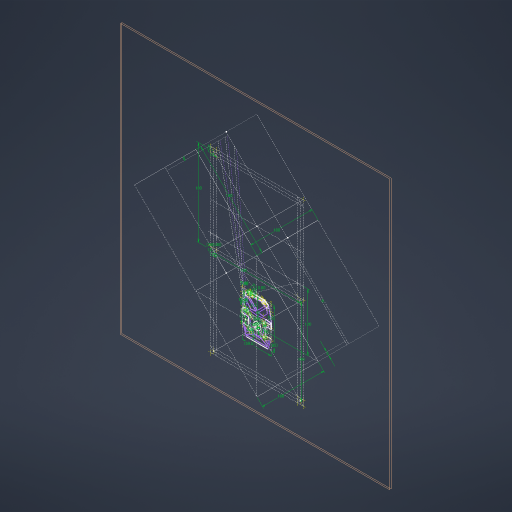
# Autodesk Inventor part: chassis
Saved by Autodesk Inventor 2023.5 (Build 275446000, 446)
## iProperties
Created: 2024-12-08
Part Number: chassis
Material: 一般
Document SubType Name: Modeling
Designer: IshiiLabHonda
Density: 1 g/cm^3
Appearance: 既定
Author: IshiiLabHonda
Autodesk Inventor part; units mm, degrees
(part 1 of 2)
ref_plane "YZ Plane" through (0, 0, 0) normal (1, 0, 0) x (0, 1, 0)
ref_plane "XZ Plane" through (0, 0, 0) normal (0, 1, 0) x (-1, 0, 0)
sketch "スケッチ1" plane through (0, 0, 0) normal (0, 0, 1) x (1, 0, 0)
  line L0 (0, 0) -> (0, 1) construction
  line L1 (0, 0) -> (1, 0) construction
  line L2 (-90, 90) -> (90, 90) construction
  line L3 (90, 90) -> (90, -90) construction
  line L4 (90, -90) -> (-90, -90) construction
  line L5 (-90, -90) -> (-90, 90) construction
  line L6 (-90, -90) -> (90, 90) construction
  line L7 (-90, 90) -> (90, -90) construction
  line L8 (-84, 96) -> (-84, 84) construction
  line L9 (-84, 84) -> (-96, 84) construction
  line L10 (-96, 84) -> (-96, 96) construction
  line L11 (-96, 96) -> (-84, 84) construction
  line L12 (-84, 96) -> (-96, 84) construction
  line L13 (-96, 96) -> (-84, 96) construction
  line L14 (-96, -96) -> (-96, -84) construction
  line L15 (-84, -96) -> (-96, -96) construction
  line L16 (-96, -96) -> (-84, -84) construction
  line L17 (-96, -84) -> (-84, -96) construction
  line L18 (-84, -84) -> (-84, -96) construction
  line L19 (-96, -84) -> (-84, -84) construction
  line L20 (96, -96) -> (84, -96) construction
  line L21 (96, -84) -> (96, -96) construction
  line L22 (96, -96) -> (84, -84) construction
  line L23 (84, -96) -> (96, -84) construction
  line L24 (84, -84) -> (96, -84) construction
  line L25 (84, -96) -> (84, -84) construction
  line L26 (96, 96) -> (96, 84) construction
  line L27 (84, 96) -> (96, 96) construction
  line L28 (96, 96) -> (84, 84) construction
  line L29 (96, 84) -> (84, 96) construction
  line L30 (84, 84) -> (84, 96) construction
  line L31 (96, 84) -> (84, 84) construction
  line L32 (-84, 84) -> (-84, -84) construction
  line L33 (-96, 84) -> (-96, -84) construction
  line L34 (-84, -84) -> (84, -84) construction
  line L35 (-84, -96) -> (84, -96) construction
  line L36 (96, 84) -> (96, -84) construction
  line L37 (84, 84) -> (84, -84) construction
  line L38 (-84, 96) -> (84, 96) construction
  line L39 (-84, 84) -> (84, 84) construction
  line L40 (-18, 15) -> (18, 15) construction
  line L41 (18, 15) -> (18, -15) construction
  line L42 (18, -15) -> (-18, -15) construction
  line L43 (-18, -15) -> (-18, 15) construction
  line L44 (-18, 15) -> (18, -15) construction
  line L45 (18, 15) -> (-18, -15) construction
  line L46 (-29.25, 11.5) -> (-18, 11.5) construction
  line L47 (-18, -11.5) -> (-29.25, -11.5) construction
  line L48 (-29.25, -11.5) -> (-29.25, 11.5) construction
  line L49 (-29.25, 11.5) -> (-18, -11.5) construction
  line L50 (-18, 11.5) -> (-29.25, -11.5) construction
  line L51 (29.25, 11.5) -> (18, 11.5) construction
  line L52 (18, -11.5) -> (29.25, -11.5) construction
  line L53 (29.25, -11.5) -> (29.25, 11.5) construction
  line L54 (29.25, 11.5) -> (18, -11.5) construction
  line L55 (18, 11.5) -> (29.25, -11.5) construction
  line L56 (-18, -10) -> (18, -10) construction
  line L57 (-18, -12.5) -> (18, -12.5) construction
  line L58 (-18, 10) -> (18, 10) construction
  line L59 (-18, 12.5) -> (18, 12.5) construction
  line L60 (-16, -15) -> (-16, 15) construction
  line L61 (16, -15) -> (16, 15) construction
  line L62 (-12, -10) -> (-12, -15) construction
  line L63 (-16, -10) -> (-12, -15) construction
  line L64 (-16, -15) -> (-12, -10) construction
  circle A0 centre (-14, -12.5) radius 0.8 construction
  line L65 (12, -10) -> (12, -15) construction
  line L66 (16, -10) -> (12, -15) construction
  line L67 (16, -15) -> (12, -10) construction
  circle A1 centre (14, -12.5) radius 0.8 construction
  line L68 (-12, 10) -> (-12, 15) construction
  line L69 (-16, 10) -> (-12, 15) construction
  line L70 (-16, 15) -> (-12, 10) construction
  circle A2 centre (-14, 12.5) radius 0.8 construction
  line L71 (12, 10) -> (12, 15) construction
  line L72 (16, 10) -> (12, 15) construction
  circle A3 centre (14, 12.5) radius 0.8 construction
  line L73 (16, 15) -> (12, 10) construction
  line L74 (-96, 276) -> (-84, 276) construction
  line L75 (-84, 276) -> (-84, 264) construction
  line L76 (-84, 264) -> (-96, 264) construction
  line L77 (-96, 264) -> (-96, 276) construction
  line L78 (-96, 276) -> (-84, 264) construction
  line L79 (-84, 276) -> (-96, 264) construction
  line L80 (-90, 90) -> (-90, 270) construction
  line L81 (-96, 264) -> (-96, 96) construction
  line L82 (-84, 264) -> (-84, 96) construction
  line L83 (96, 276) -> (84, 276) construction
  line L84 (84, 276) -> (84, 264) construction
  line L85 (84, 264) -> (96, 264) construction
  line L86 (96, 264) -> (96, 276) construction
  line L87 (96, 276) -> (84, 264) construction
  line L88 (84, 276) -> (96, 264) construction
  line L89 (90, 90) -> (90, 270) construction
  line L90 (96, 264) -> (96, 96) construction
  line L91 (84, 264) -> (84, 96) construction
  line L92 (-84, 276) -> (84, 276) construction
  line L93 (-84, 264) -> (84, 264) construction
  line L94 (-90, 270) -> (90, 270) construction
  line L95 (-90, 270) -> (90, 90) construction
  line L96 (-90, 90) -> (90, 270) construction
  circle A4 centre (0, 0) radius 15 construction
  line L97 (-96, 120) -> (96, 120) construction
  line L98 (0, 127.2792) -> (0, -127.2792) construction
  line L99 (-127.2792, 0) -> (127.2792, 0) construction
  line L100 (127.2792, 0) -> (0, -127.2792) construction
  line L101 (0, -127.2792) -> (-127.2792, 0) construction
  line L102 (-127.2792, 0) -> (0, 127.2792) construction
  line L103 (0, 127.2792) -> (127.2792, 0) construction
  line L104 (127.2792, 254.5584) -> (254.5584, 127.2792) construction
  line L105 (254.5584, 127.2792) -> (127.2792, 0) construction
  line L106 (127.2792, 0) -> (0, 127.2792) construction
  line L107 (0, 127.2792) -> (127.2792, 254.5584) construction
  line L108 (-127.2792, 254.5584) -> (0, 127.2792) construction
  line L109 (0, 127.2792) -> (-127.2792, 0) construction
  line L110 (-127.2792, 0) -> (-254.5584, 127.2792) construction
  line L111 (-254.5584, 127.2792) -> (-127.2792, 254.5584) construction
  line L112 (0, 381.8377) -> (127.2792, 254.5584) construction
  line L113 (127.2792, 254.5584) -> (0, 127.2792) construction
  line L114 (0, 127.2792) -> (-127.2792, 254.5584) construction
  line L115 (-127.2792, 254.5584) -> (0, 381.8377) construction
  line L116 (190.9188, 63.6396) -> (63.6396, 190.9188) construction
  line L117 (-190.9188, 190.9188) -> (-63.6396, 63.6396) construction
  line L118 (59.397, -59.397) -> (186.6762, 67.8823) construction
  line L119 (59.397, 186.6762) -> (186.6762, 59.397) construction
  line L120 (63.6396, 190.9188) -> (-63.6396, 318.1981) construction
  line L121 (-186.6762, 186.6762) -> (-59.397, 313.9554) construction
  point P0 (-90, -90)
  point P1 (90, -90)
  point P2 (-23.625, 0)
  point P3 (-84, 120)
  point P4 (84, 120)
  point P5 (0, 0)
  dimension "d0" = 1
  dimension "d1" = 1
  dimension "d2" = 180
  dimension "d3" = 180
  dimension "d4" = 12
  dimension "d5" = 12
  dimension "d8" = 360
  dimension "d10" = 36
  dimension "d12" = 11.25
  dimension "d13" = 23
  dimension "d14" = 5
  dimension "d15" = 2
  dimension "d16" = 4
  dimension "d17" = 1.6
  dimension "d22" = 12
  dimension "d23" = 12
  dimension "d24" = 180
  dimension "d25" = 25
  dimension "d26" = 30
  dimension "d27" = 30
  dimension "d29" = 120
  dimension "d331" = 180
  dimension "d334" = 180
  dimension "d337" = 180
  dimension "d340" = 6
  dimension "d341" = 6
  dimension "d342" = 6
  constraints: 244 end point, 29 point on line, 27 symmetric about line, 19 midpoint, 18 parallel, 10 perpendicular, 5 centre point, 4 coincident, 2 collinear, 1 horizontal, 1 vertical, 91 other
  measures "d0" distance of L0.start L0.end
  measures "d1" distance of L0.start L1.end
  measures "d2" distance of L2.start L2.end
  measures "d3" distance of L2.end L3.end
  measures "d4" distance of L9.end L10.end
  measures "d5" distance of L8.end L9.end
  measures "d10" distance of L40.start L40.end
  measures "d12" distance of L46.start L46.end
  measures "d13" distance of L47.end L46.start
  measures "d14" distance between parallel lines of L56 L42
  measures "d15" distance between parallel lines of L43 L60
  measures "d16" distance between parallel lines of L60 L62
  measures "d17" diameter of A0
  measures "d22" distance of L75.end L76.end
  measures "d23" distance of L76.end L74.start
  measures "d24" distance of L2.start L80.end
  measures "d25" distance between parallel lines of L57 L59
  measures "d26" distance between parallel lines of L42 L40
  measures "d27" diameter of A4
  measures "d29" distance between parallel lines of L1 L97
  measures "d331" distance of L100.start L100.end
  measures "d334" distance of L102.end L104.start
  measures "d337" distance of L102.end L108.start
  measures "d340" distance between parallel lines of L118 L105
  measures "d341" distance between parallel lines of L116 L119
  measures "d342" distance between parallel lines of L111 L121
sketch "スケッチ4" plane through (0, 0, 0) normal (0, 0, 1) x (1, 0, 0)
  line L0 (-84, 264) -> (-96, 264) construction
  line L1 (-90, 90) -> (-90, 270) construction
  line L2 (-96, 264) -> (-96, 96) construction
  line L3 (-96, 96) -> (-84, 96) construction
  line L4 (-84, 96) -> (-84, 84) construction
  line L5 (-84, 96) -> (-96, 84) construction
  line L6 (-96, 96) -> (-84, 84) construction
  line L7 (-84, 264) -> (-84, 96) construction
  line L8 (-84, 84) -> (-96, 84) construction
  line L9 (84, -84) -> (96, -84) construction
  line L10 (84, -96) -> (96, -84) construction
  line L11 (96, -96) -> (84, -84) construction
  line L12 (96, -84) -> (96, -96) construction
  line L13 (96, -96) -> (84, -96) construction
  line L14 (0, 0) -> (0, 1) construction
  line L15 (0, 0) -> (1, 0) construction
  line L16 (16, 15) -> (12, 10) construction
  line L17 (-96, 84) -> (-96, -84) construction
  line L18 (-84, 84) -> (-84, -84) construction
  line L19 (-90, -90) -> (-90, 90) construction
  line L20 (-90, 90) -> (90, 90) construction
  line L21 (-84, -84) -> (84, -84) construction
  line L22 (-84, -96) -> (84, -96) construction
  line L23 (-90, -90) -> (90, 90) construction
  line L24 (90, -90) -> (-90, -90) construction
  line L25 (-90, 90) -> (90, -90) construction
  line L26 (84, 84) -> (84, -84) construction
  line L27 (90, 90) -> (90, -90) construction
  line L28 (96, 84) -> (96, -84) construction
  line L29 (-96, 84) -> (-96, 96) construction
  line L30 (-84, -84) -> (-84, -96) construction
  line L31 (-96, -84) -> (-84, -84) construction
  line L32 (-84, -96) -> (-96, -96) construction
  line L33 (-96, -96) -> (-84, -84) construction
  line L34 (-96, -84) -> (-84, -96) construction
  line L35 (-96, -96) -> (-96, -84) construction
  line L36 (84, -96) -> (84, -84) construction
  line L37 (-18, -15) -> (-18, 15) construction
  line L38 (-29.25, 11.5) -> (-18, 11.5) construction
  line L39 (-18, -11.5) -> (-29.25, -11.5) construction
  line L40 (-18, 11.5) -> (-29.25, -11.5) construction
  line L41 (-29.25, 11.5) -> (-18, -11.5) construction
  line L42 (-29.25, -11.5) -> (-29.25, 11.5) construction
  line L43 (12, 10) -> (12, 15) construction
  circle A0 centre (14, 12.5) radius 0.8 construction
  line L44 (29.25, 11.5) -> (18, 11.5) construction
  line L45 (16, 10) -> (12, 15) construction
  circle A1 centre (14, -12.5) radius 0.8 construction
  line L46 (16, -15) -> (12, -10) construction
  line L47 (16, -10) -> (12, -15) construction
  line L48 (12, -10) -> (12, -15) construction
  circle A2 centre (-14, -12.5) radius 0.8 construction
  line L49 (-12, -10) -> (-12, -15) construction
  line L50 (-16, -15) -> (-12, -10) construction
  line L51 (-16, -10) -> (-12, -15) construction
  line L52 (96, 84) -> (84, 84) construction
  line L53 (96, 96) -> (96, 84) construction
  line L54 (84, 96) -> (96, 96) construction
  line L55 (96, 96) -> (84, 84) construction
  line L56 (84, 84) -> (84, 96) construction
  line L57 (96, 84) -> (84, 96) construction
  line L58 (-96, 264) -> (-96, 276) construction
  line L59 (-84, 276) -> (-84, 264) construction
  line L60 (-96, 276) -> (-84, 276) construction
  line L61 (-96, 276) -> (-84, 264) construction
  line L62 (-84, 276) -> (-96, 264) construction
  line L63 (-84, 84) -> (84, 84) construction
  line L64 (-84, 96) -> (84, 96) construction
  line L65 (84, 264) -> (84, 96) construction
  line L66 (90, 90) -> (90, 270) construction
  line L67 (-90, 90) -> (90, 270) construction
  line L68 (-90, 270) -> (90, 90) construction
  line L69 (96, 264) -> (96, 96) construction
  line L70 (-96, 120) -> (96, 120) construction
  line L71 (-84, 264) -> (84, 264) construction
  line L72 (-84, 276) -> (84, 276) construction
  line L73 (-90, 270) -> (90, 270) construction
  line L74 (84, 276) -> (84, 264) construction
  line L75 (84, 264) -> (96, 264) construction
  line L76 (96, 264) -> (96, 276) construction
  line L77 (96, 276) -> (84, 264) construction
  line L78 (96, 276) -> (84, 276) construction
  line L79 (84, 276) -> (96, 264) construction
  line L80 (-18, 15) -> (18, 15) construction
  line L81 (18, 15) -> (18, -15) construction
  line L82 (18, -15) -> (-18, -15) construction
  circle A3 centre (-14, 12.5) radius 0.8 construction
  line L83 (-16, 10) -> (-12, 15) construction
  line L84 (-12, 10) -> (-12, 15) construction
  line L85 (-16, 15) -> (-12, 10) construction
  circle A4 centre (0, 0) radius 15 construction
  line L86 (-18, 10) -> (18, 10) construction
  line L87 (-18, 12.5) -> (18, 12.5) construction
  line L88 (-18, 15) -> (18, -15) construction
  line L89 (18, 15) -> (-18, -15) construction
  line L90 (-18, -10) -> (18, -10) construction
  line L91 (-18, -12.5) -> (18, -12.5) construction
  line L92 (16, -15) -> (16, 15) construction
  line L93 (18, 11.5) -> (29.25, -11.5) construction
  line L94 (18, -11.5) -> (29.25, -11.5) construction
  line L95 (29.25, -11.5) -> (29.25, 11.5) construction
  line L96 (29.25, 11.5) -> (18, -11.5) construction
  line L97 (-16, -15) -> (-16, 15) construction
  line L98 (-84, 120) -> (29.25, 40.7015) construction
  line L99 (84, 120) -> (-29.25, 40.7015) construction
  line L100 (-29.25, 55) -> (29.25, 55) construction
  line L101 (-1.8558, 55) -> (-29.25, 35.8184) construction
  line L102 (1.8558, 55) -> (29.25, 35.8184) construction
  line L103 (-15.8034, 55) -> (-29.25, 45.5846) construction
  line L104 (-13.0898, 56.2897) -> (-9.0748, 50.5556) construction
  line L105 (-9.0748, 50.5556) -> (-14.3993, 46.8274) construction
  line L106 (-14.3993, 46.8274) -> (-18.4143, 52.5615) construction
  line L107 (-18.4143, 52.5615) -> (-13.0898, 56.2897) construction
  line L108 (-13.0898, 56.2897) -> (-14.3993, 46.8274) construction
  line L109 (-9.0748, 50.5556) -> (-18.4143, 52.5615) construction
  line L110 (-12.5162, 55.4705) -> (-17.8407, 51.7423) construction
  line L111 (-9.6483, 51.3748) -> (-14.9728, 47.6465) construction
  line L112 (-13.7445, 51.5585) -> (-13.0892, 52.0174) construction
  line L113 (-13.7445, 51.5585) -> (-13.2857, 50.9032) construction
  line L114 (-13.3762, 53.6476) -> (-11.6554, 51.1902) construction
  line L115 (-11.6554, 51.1902) -> (-14.1129, 49.4694) construction
  line L116 (-14.1129, 49.4694) -> (-15.8336, 51.9269) construction
  line L117 (-15.8336, 51.9269) -> (-13.3762, 53.6476) construction
  line L118 (-13.3762, 53.6476) -> (-14.1129, 49.4694) construction
  line L119 (-11.6554, 51.1902) -> (-15.8336, 51.9269) construction
  circle A5 centre (-13.7445, 51.5585) radius 0.8 construction
  line L120 (-29.25, 11.5) -> (-29.25, 55) construction
  line L121 (29.25, 11.5) -> (29.25, 55) construction
  line L122 (-8.9966, 50) -> (8.9966, 50) construction
  line L123 (-29.75, 55) -> (-29.75, -30) construction
  line L124 (29.75, 55) -> (29.75, -30) construction
  line L125 (-29.25, 55) -> (-29.75, 55) construction
  line L126 (29.25, 55) -> (29.75, 55) construction
  line L127 (-29.75, 8.5) -> (29.75, 8.5) construction
  line L128 (-29.75, -8.5) -> (29.75, -8.5) construction
  circle A6 centre (0, 0) radius 7.5 construction
  line L129 (-29.75, -30) -> (29.75, -30) construction
  line L130 (-29.25, 45.5846) -> (-29.75, 45.2345) construction
  line L131 (-29.25, 35.8184) -> (-29.75, 35.4683) construction
  line L132 (-25.25, 18.5) -> (-25.3613, 19.2922) construction
  line L133 (-25.25, 18.5) -> (-24.4578, 18.6113) construction
  line L134 (-28.0736, 20.6277) -> (-23.1223, 21.3236) construction
  line L135 (-23.1223, 21.3236) -> (-22.4264, 16.3723) construction
  line L136 (-22.4264, 16.3723) -> (-27.3777, 15.6764) construction
  line L137 (-27.3777, 15.6764) -> (-28.0736, 20.6277) construction
  line L138 (-28.0736, 20.6277) -> (-22.4264, 16.3723) construction
  line L139 (-23.1223, 21.3236) -> (-27.3777, 15.6764) construction
  circle A7 centre (-25.25, 18.5) radius 0.8 construction
  line L140 (-25.25, 55) -> (-25.25, -30) construction
  line L141 (-96, 180) -> (96, 180) construction
  line L142 (-25.3613, 19.2922) -> (-65.8646, 307.4878) construction
  line L143 (-186.6762, 186.6762) -> (-59.397, 313.9554) construction
  line L144 (59.397, 186.6762) -> (186.6762, 59.397) construction
  line L145 (-25.25, 18.5) -> (-80.9717, 292.3807) construction
  line L146 (-25.25, 18.5) -> (-47.5722, 302.1307) construction
  line L147 (63.6396, 190.9188) -> (-63.6396, 318.1981) construction
  line L148 (13.0898, 56.2897) -> (9.0748, 50.5556) construction
  line L149 (9.0748, 50.5556) -> (14.3993, 46.8274) construction
  line L150 (14.3993, 46.8274) -> (18.4143, 52.5615) construction
  line L151 (18.4143, 52.5615) -> (13.0898, 56.2897) construction
  line L152 (13.0898, 56.2897) -> (14.3993, 46.8274) construction
  line L153 (9.0748, 50.5556) -> (18.4143, 52.5615) construction
  line L154 (12.5162, 55.4705) -> (17.8407, 51.7423) construction
  line L155 (9.6483, 51.3748) -> (14.9728, 47.6465) construction
  line L156 (13.7445, 51.5585) -> (13.0892, 52.0174) construction
  line L157 (13.7445, 51.5585) -> (13.2857, 50.9032) construction
  line L158 (13.3762, 53.6476) -> (11.6554, 51.1902) construction
  line L159 (11.6554, 51.1902) -> (14.1129, 49.4694) construction
  line L160 (14.1129, 49.4694) -> (15.8336, 51.9269) construction
  line L161 (15.8336, 51.9269) -> (13.3762, 53.6476) construction
  line L162 (13.3762, 53.6476) -> (14.1129, 49.4694) construction
  line L163 (11.6554, 51.1902) -> (15.8336, 51.9269) construction
  circle A8 centre (13.7445, 51.5585) radius 0.8 construction
  line L164 (-23.1223, 21.3236) -> (-18.1709, 22.0195) construction
  line L165 (-18.1709, 22.0195) -> (-17.4751, 17.0681) construction
  line L166 (-17.4751, 17.0681) -> (-22.4264, 16.3723) construction
  line L167 (-23.1223, 21.3236) -> (-28.0736, 20.6277) construction
  line L168 (-28.0736, 20.6277) -> (-27.3777, 15.6764) construction
  line L169 (-27.3777, 15.6764) -> (-22.4264, 16.3723) construction
  line L170 (27.3777, 15.6764) -> (28.0736, 20.6277) construction
  line L171 (23.1223, 21.3236) -> (18.1709, 22.0195) construction
  line L172 (18.1709, 22.0195) -> (17.4751, 17.0681) construction
  line L173 (17.4751, 17.0681) -> (22.4264, 16.3723) construction
  line L174 (23.1223, 21.3236) -> (28.0736, 20.6277) construction
  line L175 (28.0736, 20.6277) -> (27.3777, 15.6764) construction
  line L176 (27.3777, 15.6764) -> (22.4264, 16.3723) construction
  line L177 (23.1223, 21.3236) -> (27.3777, 15.6764) construction
  line L178 (22.4264, 16.3723) -> (28.0736, 20.6277) construction
  line L179 (-20.2987, 19.1959) -> (-61.4376, 311.9148) construction
  line L180 (-20.2987, 19.1959) -> (-76.7397, 296.6126) construction
  line L181 (-20.2987, 19.1959) -> (-42.1385, 296.6969) construction
  line L182 (-23.1223, 21.3236) -> (-17.4751, 17.0681) construction
  line L183 (-22.4264, 16.3723) -> (-18.1709, 22.0195) construction
  point P0 (90, -90)
  point P1 (-90, -90)
  point P2 (-23.625, 0)
  point P3 (0, 61.1826)
  point P4 (-8.8296, 55)
  point P5 (-11.0823, 53.4227)
  point P6 (0, 180)
  point P7 (11.0823, 53.4227)
  dimension "d264" = 110
  dimension "d275" = 7
  dimension "d276" = 6.5
  dimension "d277" = 5
  dimension "d278" = 3
  dimension "d279" = 3
  dimension "d280" = 1.6
  dimension "d281" = 8
  dimension "d284" = 5
  dimension "d288" = 17
  dimension "d289" = 15
  dimension "d290" = 0.5
  dimension "d291" = 0.5
  dimension "d292" = 85
  dimension "d296" = 5
  dimension "d297" = 5
  dimension "d298" = 1.6
  dimension "d299" = 8
  dimension "d345" = 7
  dimension "d346" = 7
  dimension "d356" = 15
  dimension "d367" = 4
  dimension "d369" = 40
  dimension "d370" = 6
  dimension "d371" = 59.5
  dimension "d382" = 5
  dimension "d385" = 7
  constraints: 166 end point, 38 point on line, 25 symmetric about line, 18 parallel, 13 midpoint, 13 perpendicular, 6 point on circle, 5 collinear, 4 centre point, 4 coincident, 2 equal length, 8 other
  measures "d264" angle of L99 L98
  measures "d275" distance of L104.start L104.end
  measures "d276" distance of L106.end L104.start
  measures "d277" distance between parallel lines of L110 L111
  measures "d278" distance of L115.end L116.end
  measures "d279" distance of L114.end L115.end
  measures "d280" diameter of A5
  measures "d281" distance between parallel lines of L101 L103
  measures "d284" distance between parallel lines of L100 L122
  measures "d288" distance between parallel lines of L128 L127
  measures "d289" diameter of A6
  measures "d290" distance between parallel lines of L123 L120
  measures "d291" distance between parallel lines of L121 L124
  measures "d292" distance between parallel lines of L129 L100
  measures "d296" distance of L135.end L136.end
  measures "d297" distance of L134.end L135.end
  measures "d298" diameter of A7
  measures "d299" angle of L140 L132
  measures "d345" angle of L145 L146
  measures "d346" distance from line of L38 L132.start
  measures "d356" distance between parallel lines of L129 L82
  measures "d367" distance between parallel lines of L120 L140
  measures "d369" distance between parallel lines of L80 L100
  measures "d370" distance of L112.start point (-8.83, 55)
  measures "d371" distance of L123.end L124.end
  measures "d382" distance of L134.end L164.end
  measures "d385" angle of L180 L181
sketch "スケッチ5" plane through (0, 0, 0) normal (0, 0, 1) x (1, 0, 0)
  line L0 (0, 0) -> (0, 1) construction
  line L1 (29.25, 11.5) -> (18, 11.5) construction
  line L2 (18, 11.5) -> (29.25, -11.5) construction
  line L3 (29.25, 11.5) -> (18, -11.5) construction
  line L4 (29.25, -11.5) -> (29.25, 11.5) construction
  line L5 (18, -11.5) -> (29.25, -11.5) construction
  line L6 (-90, 90) -> (90, 90) construction
  line L7 (-90, -90) -> (90, 90) construction
  line L8 (-90, 90) -> (90, -90) construction
  line L9 (-84, 84) -> (-84, -84) construction
  line L10 (-96, 84) -> (-96, -84) construction
  line L11 (-90, -90) -> (-90, 90) construction
  line L12 (-84, 84) -> (-96, 84) construction
  line L13 (-96, 84) -> (-96, 96) construction
  line L14 (84, 84) -> (84, -84) construction
  line L15 (90, 90) -> (90, -90) construction
  line L16 (96, 84) -> (84, 84) construction
  line L17 (96, 84) -> (96, -84) construction
  line L18 (90, -90) -> (-90, -90) construction
  line L19 (-84, -84) -> (84, -84) construction
  line L20 (-84, -96) -> (84, -96) construction
  line L21 (-84, -84) -> (-84, -96) construction
  line L22 (-96, -96) -> (-96, -84) construction
  line L23 (-84, -96) -> (-96, -96) construction
  line L24 (-96, -96) -> (-84, -84) construction
  line L25 (-96, -84) -> (-84, -96) construction
  line L26 (-96, -84) -> (-84, -84) construction
  line L27 (0, 0) -> (1, 0) construction
  line L28 (-84, 264) -> (-96, 264) construction
  line L29 (-96, 276) -> (-84, 276) construction
  line L30 (-96, 264) -> (-96, 276) construction
  line L31 (-84, 276) -> (-96, 264) construction
  line L32 (-96, 276) -> (-84, 264) construction
  line L33 (-84, 276) -> (-84, 264) construction
  line L34 (84, -96) -> (84, -84) construction
  line L35 (96, -96) -> (84, -96) construction
  line L36 (96, -84) -> (96, -96) construction
  line L37 (96, -96) -> (84, -84) construction
  line L38 (84, -96) -> (96, -84) construction
  line L39 (84, -84) -> (96, -84) construction
  line L40 (-18, 15) -> (18, 15) construction
  line L41 (18, 15) -> (18, -15) construction
  line L42 (16, 15) -> (12, 10) construction
  line L43 (12, 10) -> (12, 15) construction
  line L44 (16, 10) -> (12, 15) construction
  line L45 (16, -15) -> (16, 15) construction
  line L46 (-18, 10) -> (18, 10) construction
  line L47 (-18, 12.5) -> (18, 12.5) construction
  circle A0 centre (0, 0) radius 15 construction
  line L48 (-18, -10) -> (18, -10) construction
  line L49 (-18, -12.5) -> (18, -12.5) construction
  line L50 (18, -15) -> (-18, -15) construction
  line L51 (-18, 15) -> (18, -15) construction
  line L52 (18, 15) -> (-18, -15) construction
  line L53 (-16, -15) -> (-16, 15) construction
  line L54 (-18, -15) -> (-18, 15) construction
  line L55 (-29.25, 11.5) -> (-18, 11.5) construction
  line L56 (-18, -11.5) -> (-29.25, -11.5) construction
  line L57 (-29.25, -11.5) -> (-29.25, 11.5) construction
  line L58 (-29.25, 11.5) -> (-18, -11.5) construction
  line L59 (-18, 11.5) -> (-29.25, -11.5) construction
  line L60 (-12, 10) -> (-12, 15) construction
  circle A1 centre (-14, 12.5) radius 0.8 construction
  line L61 (-16, 10) -> (-12, 15) construction
  line L62 (-16, 15) -> (-12, 10) construction
  circle A2 centre (14, 12.5) radius 0.8 construction
  line L63 (-84, 96) -> (-96, 84) construction
  line L64 (-96, 96) -> (-84, 96) construction
  line L65 (-84, 96) -> (-84, 84) construction
  line L66 (-96, 96) -> (-84, 84) construction
  line L67 (-96, 264) -> (-96, 96) construction
  line L68 (-84, 264) -> (-84, 96) construction
  line L69 (-84, 96) -> (84, 96) construction
  line L70 (-84, 84) -> (84, 84) construction
  line L71 (84, 84) -> (84, 96) construction
  line L72 (96, 96) -> (96, 84) construction
  line L73 (96, 96) -> (84, 84) construction
  line L74 (96, 84) -> (84, 96) construction
  line L75 (-96, 120) -> (96, 120) construction
  line L76 (84, 96) -> (96, 96) construction
  line L77 (-84, 264) -> (84, 264) construction
  line L78 (84, 264) -> (84, 96) construction
  line L79 (-84, 276) -> (84, 276) construction
  line L80 (96, 264) -> (96, 96) construction
  line L81 (-90, 270) -> (90, 270) construction
  line L82 (-90, 270) -> (90, 90) construction
  line L83 (-90, 90) -> (90, 270) construction
  line L84 (90, 90) -> (90, 270) construction
  line L85 (-90, 90) -> (-90, 270) construction
  line L86 (84, 264) -> (96, 264) construction
  line L87 (96, 276) -> (84, 276) construction
  line L88 (96, 276) -> (84, 264) construction
  line L89 (84, 276) -> (96, 264) construction
  line L90 (96, 264) -> (96, 276) construction
  line L91 (84, 276) -> (84, 264) construction
  circle A3 centre (-14, -12.5) radius 0.8 construction
  line L92 (-12, -10) -> (-12, -15) construction
  line L93 (-16, -15) -> (-12, -10) construction
  line L94 (12, -10) -> (12, -15) construction
  circle A4 centre (14, -12.5) radius 0.8 construction
  line L95 (16, -15) -> (12, -10) construction
  line L96 (16, -10) -> (12, -15) construction
  line L97 (-16, -10) -> (-12, -15) construction
  line L98 (-15.8336, 51.9269) -> (-13.3762, 53.6476) construction
  line L99 (-11.6554, 51.1902) -> (-15.8336, 51.9269) construction
  circle A5 centre (-13.7445, 51.5585) radius 0.8 construction
  line L100 (-11.6554, 51.1902) -> (-14.1129, 49.4694) construction
  line L101 (-13.3762, 53.6476) -> (-14.1129, 49.4694) construction
  line L102 (-14.1129, 49.4694) -> (-15.8336, 51.9269) construction
  line L103 (-29.25, 45.5846) -> (-29.75, 45.2345) construction
  line L104 (-15.8034, 55) -> (-29.25, 45.5846) construction
  line L105 (-29.25, 55) -> (-29.75, 55) construction
  line L106 (-13.3762, 53.6476) -> (-11.6554, 51.1902) construction
  line L107 (-29.25, 55) -> (29.25, 55) construction
  line L108 (-9.0748, 50.5556) -> (-14.3993, 46.8274) construction
  line L109 (-14.3993, 46.8274) -> (-18.4143, 52.5615) construction
  line L110 (-13.0898, 56.2897) -> (-9.0748, 50.5556) construction
  line L111 (-1.8558, 55) -> (-29.25, 35.8184) construction
  line L112 (1.8558, 55) -> (29.25, 35.8184) construction
  line L113 (-18, 15) -> (18, 15) construction
  line L114 (12, 10) -> (12, 15) construction
  line L115 (-18, 10) -> (18, 10) construction
  circle A6 centre (-14, 12.5) radius 0.8 construction
  line L116 (-12, 10) -> (-12, 15) construction
  line L117 (-16, 10) -> (-12, 15) construction
  line L118 (-16, 15) -> (-12, 10) construction
  line L119 (-18, 12.5) -> (18, 12.5) construction
  line L120 (29.25, 55) -> (29.75, 55) construction
  line L121 (29.25, 11.5) -> (29.25, 55) construction
  line L122 (-8.9966, 50) -> (8.9966, 50) construction
  line L123 (-29.25, 35.8184) -> (-29.75, 35.4683) construction
  line L124 (-29.25, 11.5) -> (-29.25, 55) construction
  line L125 (-9.6483, 51.3748) -> (-14.9728, 47.6465) construction
  line L126 (-13.7445, 51.5585) -> (-13.2857, 50.9032) construction
  line L127 (-13.7445, 51.5585) -> (-13.0892, 52.0174) construction
  line L128 (-9.0748, 50.5556) -> (-18.4143, 52.5615) construction
  line L129 (-12.5162, 55.4705) -> (-17.8407, 51.7423) construction
  line L130 (-18.4143, 52.5615) -> (-13.0898, 56.2897) construction
  line L131 (-13.0898, 56.2897) -> (-14.3993, 46.8274) construction
  line L132 (-29.25, 11.5) -> (-18, 11.5) construction
  line L133 (-29.25, 11.5) -> (-18, -11.5) construction
  line L134 (29.25, 11.5) -> (18, 11.5) construction
  line L135 (29.25, -11.5) -> (29.25, 11.5) construction
  line L136 (18, 11.5) -> (29.25, -11.5) construction
  line L137 (29.25, 11.5) -> (18, -11.5) construction
  line L138 (0, 0) -> (0, 1) construction
  line L139 (0, 0) -> (1, 0) construction
  circle A7 centre (0, 0) radius 7.5 construction
  circle A8 centre (0, 0) radius 15 construction
  line L140 (-16, -15) -> (-16, 15) construction
  circle A9 centre (14, 12.5) radius 0.8 construction
  line L141 (-12, -10) -> (-12, -15) construction
  line L142 (12, -10) -> (12, -15) construction
  line L143 (16, 10) -> (12, 15) construction
  line L144 (-16, -15) -> (-12, -10) construction
  line L145 (16, -10) -> (12, -15) construction
  line L146 (16, 15) -> (12, 10) construction
  line L147 (-18, -12.5) -> (18, -12.5) construction
  line L148 (18, -15) -> (-18, -15) construction
  line L149 (-18, 11.5) -> (-29.25, -11.5) construction
  line L150 (18, -11.5) -> (29.25, -11.5) construction
  line L151 (-18, -11.5) -> (-29.25, -11.5) construction
  line L152 (-29.25, -11.5) -> (-29.25, 11.5) construction
  line L153 (16, -15) -> (16, 15) construction
  line L154 (18, 15) -> (18, -15) construction
  line L155 (-18, -15) -> (-18, 15) construction
  line L156 (-18, 15) -> (18, -15) construction
  line L157 (18, 15) -> (-18, -15) construction
  line L158 (-29.75, -8.5) -> (29.75, -8.5) construction
  line L159 (-29.75, 8.5) -> (29.75, 8.5) construction
  line L160 (-29.75, -30) -> (29.75, -30) construction
  line L161 (-29.75, 55) -> (-29.75, -30) construction
  line L162 (29.75, 55) -> (29.75, -30) construction
  line L163 (84, -84) -> (96, -84) construction
  line L164 (84, -96) -> (96, -84) construction
  line L165 (96, -96) -> (84, -84) construction
  line L166 (96, -84) -> (96, -96) construction
  line L167 (96, -96) -> (84, -96) construction
  line L168 (-96, 84) -> (-96, -84) construction
  line L169 (-84, 84) -> (-84, -84) construction
  line L170 (-90, -90) -> (-90, 90) construction
  line L171 (-84, -84) -> (84, -84) construction
  line L172 (-84, -96) -> (84, -96) construction
  line L173 (-90, -90) -> (90, 90) construction
  line L174 (90, -90) -> (-90, -90) construction
  line L175 (-90, 90) -> (90, -90) construction
  line L176 (84, 84) -> (84, -84) construction
  line L177 (90, 90) -> (90, -90) construction
  line L178 (96, 84) -> (96, -84) construction
  line L179 (84, -96) -> (84, -84) construction
  line L180 (-18, -10) -> (18, -10) construction
  circle A10 centre (14, -12.5) radius 0.8 construction
  line L181 (16, -15) -> (12, -10) construction
  line L182 (-16, -10) -> (-12, -15) construction
  line L183 (-84, -84) -> (-84, -96) construction
  line L184 (-96, -84) -> (-84, -84) construction
  line L185 (-84, -96) -> (-96, -96) construction
  line L186 (-96, -96) -> (-84, -84) construction
  line L187 (-96, -84) -> (-84, -96) construction
  line L188 (-96, -96) -> (-96, -84) construction
  circle A11 centre (-14, -12.5) radius 0.8 construction
  line L189 (-96, 96) -> (-84, 96) construction
  line L190 (-84, 96) -> (-84, 84) construction
  line L191 (-84, 96) -> (-96, 84) construction
  line L192 (-96, 96) -> (-84, 84) construction
  line L193 (84, 96) -> (96, 96) construction
  line L194 (96, 84) -> (84, 84) construction
  line L195 (96, 96) -> (96, 84) construction
  line L196 (96, 96) -> (84, 84) construction
  line L197 (96, 84) -> (84, 96) construction
  line L198 (-96, 120) -> (96, 120) construction
  line L199 (-84, 96) -> (84, 96) construction
  line L200 (-90, 90) -> (90, 90) construction
  line L201 (-84, 84) -> (-96, 84) construction
  line L202 (-96, 84) -> (-96, 96) construction
  line L203 (-84, 84) -> (84, 84) construction
  line L204 (84, 120) -> (-29.25, 40.7015) construction
  line L205 (-84, 120) -> (29.25, 40.7015) construction
  line L206 (84, 84) -> (84, 96) construction
  line L207 (-84, 264) -> (-96, 264) construction
  line L208 (-90, 90) -> (-90, 270) construction
  line L209 (-96, 264) -> (-96, 96) construction
  line L210 (-84, 264) -> (-84, 96) construction
  line L211 (96, 264) -> (96, 96) construction
  line L212 (84, 264) -> (84, 96) construction
  line L213 (90, 90) -> (90, 270) construction
  line L214 (-90, 90) -> (90, 270) construction
  line L215 (-90, 270) -> (90, 90) construction
  line L216 (-84, 264) -> (84, 264) construction
  line L217 (-90, 270) -> (90, 270) construction
  line L218 (-96, 264) -> (-96, 276) construction
  line L219 (-96, 276) -> (-84, 276) construction
  line L220 (-96, 276) -> (-84, 264) construction
  line L221 (-84, 276) -> (-96, 264) construction
  line L222 (-84, 276) -> (-84, 264) construction
  line L223 (-84, 276) -> (84, 276) construction
  line L224 (84, 264) -> (96, 264) construction
  line L225 (96, 264) -> (96, 276) construction
  line L226 (96, 276) -> (84, 264) construction
  line L227 (96, 276) -> (84, 276) construction
  line L228 (84, 276) -> (96, 264) construction
  line L229 (84, 276) -> (84, 264) construction
  line L230 (-29.75, 8.5) -> (-18, 8.5)
  line L231 (-29.75, -8.5) -> (-18, -8.5)
  line L232 (-18, 8.5) -> (-18, -8.5)
  line L233 (-15.8034, 55) -> (-8.8296, 55)
  line L234 (-29.75, 45.2345) -> (-29.25, 45.5846)
  line L235 (-23.7807, 49.4143) -> (-15.8034, 55)
  line L236 (-8.8296, 55) -> (8.8296, 55)
  line L237 (-8.9966, 50) -> (8.9966, 50)
  line L238 (8.9966, 50) -> (16.3936, 44.8205)
  line L239 (-16.3936, 44.8205) -> (-8.9966, 50)
  circle A12 centre (0, 0) radius 7.5
  line L240 (29.75, 8.5) -> (18, 8.5)
  line L241 (29.75, -8.5) -> (18, -8.5)
  line L242 (18, 8.5) -> (18, -8.5)
  line L243 (29.75, 8.5) -> (29.75, 8.5)
  line L244 (23.7807, 49.4143) -> (15.8034, 55)
  line L245 (8.8296, 55) -> (15.8034, 55)
  line L246 (-16.3936, 44.8205) -> (0, 28.4269)
  line L247 (16.3936, 44.8205) -> (0, 28.4269)
  line L248 (-19.3049, 42.7821) -> (-21.2944, 33.4219)
  line L249 (-19.3049, 42.7821) -> (-2.1213, 25.5985)
  line L250 (-13.256, 24.3963) -> (-2.1213, 25.5985)
  line L251 (-21.2944, 33.4219) -> (-13.256, 24.3963)
  line L252 (19.3049, 42.7821) -> (21.2944, 33.4219)
  line L253 (19.3049, 42.7821) -> (2.1213, 25.5985)
  line L254 (13.256, 24.3963) -> (2.1213, 25.5985)
  line L255 (21.2944, 33.4219) -> (13.256, 24.3963)
  line L256 (-20.895, -26.9322) -> (20.895, -26.9322)
  line L257 (20.895, -26.9322) -> (21.4865, -25.218)
  line L258 (-21.4865, -25.218) -> (-20.895, -26.9322)
  line L259 (-29.75, -8.5) -> (-22.3317, -30)
  line L260 (-22.3317, -30) -> (22.3317, -30)
  line L261 (29.75, -8.5) -> (22.3317, -30)
  line L262 (-21.4865, -25.218) -> (-6.8217, -17.6764)
  line L263 (-6.8217, -17.6764) -> (6.8217, -17.6764)
  line L264 (6.8217, -17.6764) -> (21.4865, -25.218)
  circle A13 centre (-14, 12.5) radius 1
  circle A14 centre (14, 12.5) radius 1
  circle A15 centre (-14, -12.5) radius 1
  circle A16 centre (14, -12.5) radius 1
  line L265 (-13.3762, 53.6476) -> (-15.8336, 51.9269)
  line L266 (-15.8336, 51.9269) -> (-14.1129, 49.4694)
  line L267 (-14.1129, 49.4694) -> (-11.6554, 51.1902)
  line L268 (-11.6554, 51.1902) -> (-13.3762, 53.6476)
  line L269 (-25.25, 18.5) -> (-25.3613, 19.2922) construction
  line L270 (-25.25, 18.5) -> (-24.4578, 18.6113) construction
  circle A17 centre (-25.25, 18.5) radius 0.8 construction
  line L271 (-23.1223, 21.3236) -> (-22.4264, 16.3723) construction
  line L272 (-27.3777, 15.6764) -> (-28.0736, 20.6277) construction
  line L273 (-23.1223, 21.3236) -> (-27.3777, 15.6764) construction
  line L274 (-28.0736, 20.6277) -> (-23.1223, 21.3236) construction
  line L275 (-22.4264, 16.3723) -> (-27.3777, 15.6764) construction
  line L276 (-28.0736, 20.6277) -> (-22.4264, 16.3723) construction
  line L277 (13.3762, 53.6476) -> (15.8336, 51.9269)
  line L278 (15.8336, 51.9269) -> (14.1129, 49.4694)
  line L279 (14.1129, 49.4694) -> (11.6554, 51.1902)
  line L280 (11.6554, 51.1902) -> (13.3762, 53.6476)
  line L281 (-23.7807, 49.4143) -> (-29.75, 21.3308)
  line L282 (-29.75, 21.3308) -> (-29.75, 8.5)
  line L283 (23.7807, 49.4143) -> (29.75, 21.3308)
  line L284 (29.75, 21.3308) -> (29.75, 8.5)
  line L285 (-28.0736, 20.6277) -> (-27.3777, 15.6764)
  line L286 (-25.6517, -13.5042) -> (-23.113, -20.862)
  line L287 (-23.113, -20.862) -> (-16.8015, -17.6162)
  line L288 (-16.8015, -17.6162) -> (-25.6517, -13.5042)
  line L289 (25.6517, -13.5042) -> (23.113, -20.862)
  line L290 (23.113, -20.862) -> (16.8015, -17.6162)
  line L291 (16.8015, -17.6162) -> (25.6517, -13.5042)
  line L292 (-23.1223, 21.3236) -> (-18.1709, 22.0195) construction
  line L293 (-18.1709, 22.0195) -> (-17.4751, 17.0681) construction
  line L294 (-17.4751, 17.0681) -> (-22.4264, 16.3723) construction
  line L295 (27.3777, 15.6764) -> (22.4264, 16.3723) construction
  line L296 (17.4751, 17.0681) -> (22.4264, 16.3723) construction
  line L297 (18.1709, 22.0195) -> (17.4751, 17.0681) construction
  line L298 (23.1223, 21.3236) -> (18.1709, 22.0195) construction
  line L299 (23.1223, 21.3236) -> (28.0736, 20.6277) construction
  line L300 (28.0736, 20.6277) -> (27.3777, 15.6764) construction
  line L301 (-28.0736, 20.6277) -> (-18.1709, 22.0195)
  line L302 (-17.4751, 17.0681) -> (-18.1709, 22.0195)
  line L303 (-17.4751, 17.0681) -> (-27.3777, 15.6764)
  line L304 (18.1709, 22.0195) -> (28.0736, 20.6277)
  line L305 (27.3777, 15.6764) -> (28.0736, 20.6277)
  line L306 (27.3777, 15.6764) -> (17.4751, 17.0681)
  line L307 (18.1709, 22.0195) -> (17.4751, 17.0681)
  point P0 (-90, -90)
  point P1 (90, -90)
  point P2 (-23.625, 0)
  point P3 (-11.0823, 53.4227)
  point P4 (-8.8296, 55)
  point P5 (0, 61.1826)
  point P6 (-23.625, 0)
  point P7 (-90, -90)
  point P8 (90, -90)
  point P9 (29.75, 8.5)
  dimension "d352" = 15
  dimension "d354" = 3.5
  dimension "d359" = 2
  dimension "d360" = 2
  dimension "d361" = 2
  dimension "d362" = 2
  dimension "d368" = 12
  constraints: 122 end point, 24 horizontal alignment, 14 point on line, 7 parallel, 7 perpendicular, 5 centre point, 5 coincident, 5 collinear, 1 equal length, 1 horizontal, 40 other
  measures "d352" diameter of A12
  measures "d354" distance between parallel lines of L246 L249
  measures "d359" diameter of A13
  measures "d360" diameter of A14
  measures "d361" diameter of A15
  measures "d362" diameter of A16
  measures "d368" angle of L161 L281